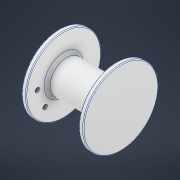
# Autodesk Inventor part: secureingReel
Saved by Autodesk Inventor 2021 (Build 250183000, 183)
## iProperties
Created: 2021-06-22
Part Number: secureingReel
Material: Aluminum 6061
Document SubType Name: Modeling
Designer: Watchdog
Density: 2.7 g/cm^3
Appearance: Aluminum - Flat
Author: Watchdog
Autodesk Inventor part; units mm, degrees
ref_plane "YZ Plane" through (0, 0, 0) normal (1, 0, 0) x (0, 1, 0)
ref_plane "XZ Plane" through (0, 0, 0) normal (0, 1, 0) x (-1, 0, 0)
ref_plane "XY Plane" through (0, 0, 0) normal (0, 0, 1) x (1, 0, 0)
sketch "Sketch1" plane through (0, 0, 0) normal (0, 0, 1) x (1, 0, 0)
  line L0 (-20.5, 25) -> (-17.5, 25)
  line L1 (-17.5, 25) -> (-17.5, 11)
  line L2 (-17.5, 11) -> (0, 11)
  line L3 (0, 11) -> (0, 0)
  line L4 (0, 0) -> (-20.5, 0)
  line L5 (-20.5, 0) -> (-20.5, 25)
  line L6 (0, 17.0507) -> (0, -8.2074)
  line L7 (20.5, 25) -> (17.5, 25)
  line L8 (17.5, 25) -> (17.5, 11)
  line L9 (17.5, 11) -> (0, 11)
  line L10 (0, 0) -> (20.5, 0)
  line L11 (20.5, 0) -> (20.5, 25)
  dimension "d0" = 3
  dimension "d1" = 11
  dimension "d2" = 25
  dimension "d3" = 17.5
  constraints: 24 end point, 4 perpendicular, 4 symmetric about line, 2 vertical, 1 horizontal, 1 point on line
  measures "d0" distance between parallel lines of L1 L5
  measures "d1" distance between parallel lines of L4 L2
  measures "d2" distance between parallel lines of L4 L0
  measures "d3" distance from line of L3.end L1
revolve "Revolution1" add sketch "Sketch1" angle 360 about axis through (0, 0, 0) along (1, 0, 0)
sketch "Sketch2" plane through (-17.5, 0, 0) normal (1, 0, 0) x (0, 0, -1)
  circle A0 centre (0, 0) radius 11 projected
  line L0 (0, 0) -> (-17.5, 0)
  line L1 (0, 0) -> (-12.3744, -12.3744)
  dimension "d23" = 17.5
  dimension "d24" = 17.5
  dimension "d25" = 45
  constraints: 4 end point, 2 coincident, 1 horizontal
  measures "d23" distance of L0.start L0.end
  measures "d24" distance of L0.start L1.end
  measures "d25" angle of L1 L0
hole "Hole1" at (-17.5, 0, 17.5) at (-17.5, -12.3744, 12.3744) direction (-1, 0, 0) diameter 3 depth 3
sketch "Sketch3" plane through (-20.5, 0, 0) normal (-1, 0, 0) x (0, 0, 1)
  circle A0 centre (0, 0) radius 3.5
  line L0 (3.1623, 1.5) -> (4.4623, 1.5)
  line L1 (4.4623, 1.5) -> (4.4623, -1.5)
  line L2 (4.4623, -1.5) -> (3.1623, -1.5)
  line L3 (3.1623, -1.5) -> (3.1623, 1.5)
  point P0 (0, 0)
  dimension "d12" = 7
  dimension "d13" = 3
  dimension "d14" = 1.3
  constraints: 8 end point, 2 parallel, 2 point on circle, 1 centre point, 1 coincident, 1 horizontal, 1 perpendicular
  measures "d12" diameter of A0
  measures "d13" distance between parallel lines of L2 L0
  measures "d14" distance between parallel lines of L3 L1
extrude "Extrusion1" cut sketch "Sketch3" against normal blind 22
chamfer "Chamfer1" distance 0.5 angle 45 4 edges at (-20.5, 0, -3.5) (-20.5, 1.5, 3.8123) (-20.5, 0, 4.4623) (-20.5, -1.5, 3.8123)
fillet "Fillet1" radius 2 2 edges at (-17.5, -11, 0) (17.5, -11, 0)
fillet "Fillet2" radius 0.5 4 edges at (-20.5, -25, 0) (-17.5, -25, 0) (17.5, -25, 0) (20.5, -25, 0)
equation "\"d0\" = tedge"
equation "\"d1\" = r1"
equation "\"d2\" = r2"
equation "\"d3\" = 0.5 * win"
equation "\"tedge\" = 3"
equation "\"r1\" = 11"
equation "\"r2\" = 25"
equation "\"win\" = 35"
body "Solid1"
